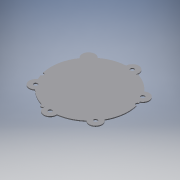
# Autodesk Inventor part: Base_bottom
Saved by Autodesk Inventor 2016 (Build 200138000, 138)
## iProperties
Created: 2015-10-08
Part Number: Base_bottom
Material: Generic
Document SubType Name: Modeling
Designer: powasar16
Density: 1 g/cm^3
Appearance: Default
Author: powasar16
Autodesk Inventor part; units mm, degrees
ref_plane "YZ Plane" through (0, 0, 0) normal (1, 0, 0) x (0, 1, 0)
ref_plane "XZ Plane" through (0, 0, 0) normal (0, 1, 0) x (-1, 0, 0)
ref_plane "XY Plane" through (0, 0, 0) normal (0, 0, 1) x (1, 0, 0)
sketch "Sketch1" plane through (0, 0, 0) normal (0, 1, 0) x (-1, 0, 0)
  arc A0 (45.4572, -61.1563) -> (62.9817, -42.8923) centre (54.9831, -52.757) ccw
  circle A1 centre (54.9831, -52.757) radius 3.75
  circle A2 centre (73.1804, 21.2382) radius 3.75 construction
  circle A3 centre (18.1974, 73.9952) radius 3.75 construction
  circle A4 centre (-54.9831, 52.757) radius 3.75 construction
  circle A5 centre (-73.1804, -21.2382) radius 3.75 construction
  circle A6 centre (-18.1974, -73.9952) radius 3.75 construction
  arc A7 (62.9817, -42.8923) -> (72.047, 24.8128) centre (0, 0) ccw
  arc A8 (-66.4803, 37.2399) -> (-72.047, -24.8128) centre (0, 0) ccw
  arc A9 (-20.846, -73.2932) -> (4.312, -76.0779) centre (-8.3834, -75.7374) ccw
  arc A10 (-70.8376, -28.0798) -> (-57.7316, -49.7343) centre (-65.19, -39.455) ccw
  arc A11 (-50.6143, 56.9617) -> (-66.4803, 37.2399) centre (-59.3719, 47.7642) ccw
  arc A12 (14.3787, 74.8311) -> (-10.9263, 75.4126) centre (1.7505, 76.1799) ccw
  arc A13 (68.1207, 34.1469) -> (53.1773, 54.5767) centre (61.5032, 44.9866) ccw
  circle A14 centre (-8.3834, -75.7374) radius 3.75
  circle A15 centre (-65.19, -39.455) radius 3.75
  circle A16 centre (-59.3719, 47.7642) radius 3.75
  circle A17 centre (1.7505, 76.1799) radius 3.75
  circle A18 centre (61.5032, 44.9866) radius 3.75
  arc A19 (-14.535, -74.8009) -> (-12.0993, -75.2333) centre (0, 0) ccw
  arc A20 (4.312, -76.0779) -> (45.4572, -61.1563) centre (0, 0) ccw
  arc A21 (-72.047, -24.8128) -> (-70.8376, -28.0798) centre (0, 0) ccw
  arc A22 (-57.7316, -49.7343) -> (-20.846, -73.2932) centre (0, 0) ccw
  arc A23 (14.535, 74.8009) -> (14.3787, 74.8311) centre (0, 0) ccw
  arc A24 (-10.9263, 75.4126) -> (-50.6143, 56.9617) centre (0, 0) ccw
  arc A25 (72.047, 24.8128) -> (68.1207, 34.1469) centre (0, 0) ccw
  arc A26 (53.1773, 54.5767) -> (14.535, 74.8009) centre (0, 0) ccw
  point P0 (73.9952, -18.1974)
  dimension "d7" = 25.4
  dimension "d15" = 7.5
  dimension "d18" = 360
  dimension "d22" = 52.5
  dimension "d23" = 80
  dimension "d24" = 52.5
  dimension "d25" = 52.5
  dimension "d26" = 52.5
  dimension "d27" = 70
  constraints: 34 point on circle, 22 centre point, 9 equal radius, 7 coincident, 39 other
  measures "d7" diameter of A0
  measures "d15" diameter of A1
extrude "Extrusion1" add sketch "Sketch1" along normal blind 1.905
body "Solid1"
